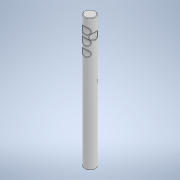
# Autodesk Inventor part: 79. Шток третьей и четвертой передач
Saved by Autodesk Inventor 2021 (Build 250183000, 183)
## iProperties
Created: 2021-03-18
Part Number: 79. Шток третьей и четвертой передач
Material: Типовые
Document SubType Name: Modeling
Designer: Данил
Density: 1 g/cm^3
Appearance: По умолчанию
Author: Данил
Autodesk Inventor part; units mm, degrees
ref_plane "YZ Plane" through (0, 0, 0) normal (1, 0, 0) x (0, 1, 0)
ref_plane "XZ Plane" through (0, 0, 0) normal (0, 1, 0) x (-1, 0, 0)
ref_plane "XY Plane" through (0, 0, 0) normal (0, 0, 1) x (1, 0, 0)
sketch "Эскиз1" plane through (0, 0, 0) normal (0, 0, 1) x (1, 0, 0)
  line L0 (0, 91.5) -> (0, -91.5)
  line L1 (0, -91.5) -> (6.75, -91.5)
  line L2 (7.5, -90.75) -> (7.5, 90.75)
  line L3 (6.75, 91.5) -> (0, 91.5)
  line L4 (7.5, -90.75) -> (6.75, -91.5)
  line L5 (7.5, 90.75) -> (6.75, 91.5)
  point P0 (0, 0)
  point P1 (0, 0)
  point P2 (7.5, -91.5)
  point P3 (7.5, 91.5)
  dimension "d0" = 183
  dimension "d1" = 15
  dimension "d2" = 0.75
  dimension "d3" = 45
  dimension "d4" = 0.75
  dimension "d5" = 45
  constraints: 12 end point, 4 point on line, 2 perpendicular, 1 coincident, 1 horizontal, 1 midpoint, 1 vertical
  measures "d0" distance of L0.start L0.end
  measures "d1" diameter of L2 L0
  measures "d2" distance of L2.start point (7.5, -91.5)
  measures "d3" angle of L2 L4
  measures "d4" distance of L2.end point (7.5, 91.5)
  measures "d5" angle of L2 L5
revolve "Вращение1" add sketch "Эскиз1" angle 360 about axis through (0, 91.5, 0) along (0, -1, 0)
sketch "Эскиз2" plane through (0, 0, 0) normal (1, 0, 0) x (0, 1, 0)
  line L0 (90.75, -7.5) -> (-90.75, -7.5) projected
  line L1 (90.75, 7.5) -> (-90.75, 7.5) projected
  line L2 (91.5, 6.75) -> (91.5, -6.75) projected
  arc A0 (71.1872, 7.5) -> (79.8128, 7.5) centre (75.5, 9.1) ccw
  arc A1 (57.6872, 7.5) -> (66.3128, 7.5) centre (62, 9.1) ccw
  arc A2 (44.1872, 7.5) -> (52.8128, 7.5) centre (48.5, 9.1) ccw
  point P0 (0, 0)
  point P1 (75.5, 4.5)
  point P2 (62, 4.5)
  point P3 (48.5, 4.5)
  point P4 (62, 4.5)
  point P5 (48.5, 4.5)
  dimension "d7" = 4.6
  dimension "d8" = 12
  dimension "d9" = 16
  dimension "d10" = 13.5
  dimension "d11" = 13.5
  constraints: 11 point on circle, 6 point on line, 4 horizontal alignment, 3 centre point, 3 vertical alignment
  measures "d7" radius of A0
  measures "d8" distance from line of L0 point (75.5, 4.5)
  measures "d9" distance from line of L2 A0.centre
  measures "d10" distance of A1.centre A0.centre
  measures "d11" distance of A2.centre A1.centre
extrude "Выдавливание1" cut sketch "Эскиз2" against normal through all both and the other way through all
ref_plane "РабПлоскость1" through (0, 10.75, 0) normal (0, 1, 0) x (1, 0, 0)
sketch "Эскиз3" plane through (0, 10.75, 0) normal (0, 1, 0) x (1, 0, 0)
  line L0 (2.0673, 7.2095) -> (-2.0673, -7.2095) construction
  circle A0 centre (0, 0) radius 7.5 projected
  line L1 (0, 0) -> (0, 7.5) construction
  point P0 (0, 0)
  point P1 (0, 0)
  dimension "d15" = 16
  constraints: 4 end point, 2 point on circle, 1 coincident, 1 midpoint, 1 vertical
  measures "d15" angle of L1 L0
ref_plane "РабПлоскость2" through (2.0673, 10.75, -7.2095) normal (-0.2756374, 0, 0.9612617) x (0, -1, 0)
hole "Отверстие1" at (2.0673, 10.75, -7.2095) direction (-0.2756374, 0, 0.9612617) diameter 4.5 depth 11 tip angle 120 countersink diameter 8.7 countersink angle 30
sketch "Эскиз4" plane through (0, 0, 0) normal (0, 0, 1) x (1, 0, 0)
  line L0 (7.5, 90.75) -> (7.5, -90.75) projected
  line L1 (-7.5, 90.75) -> (-7.5, -90.75) projected
  line L2 (-6.75, 91.5) -> (6.75, 91.5) projected
  arc A0 (7.5, 73.1997) -> (7.5, 64.3003) centre (9.3, 68.75) ccw
  ellipse E0 centre (-0.093, 10.75) end of major axis (-0.093, 8.5) minor radius 2.1628 projected
  point P0 (0, 0)
  point P1 (4.5, 68.75)
  dimension "d25" = 4.8
  dimension "d26" = 12
  dimension "d27" = 58
  constraints: 3 point on circle, 2 point on line, 1 centre point, 1 horizontal alignment
  measures "d25" radius of A0
  measures "d26" distance from line of L1 point (4.5, 68.75)
  measures "d27" vertical distance of A0.centre E0.centre
extrude "Выдавливание2" cut sketch "Эскиз4" along normal through all both and the other way through all contours L0 A0
mirror "Зеркальное отражение1" about plane through (0, 0, 0) normal (1, 0, 0) of "Выдавливание2"
fillet "Сопряжение1" radius 0.8 13 edges at (-4.2073, 79.0778, 6.2087) (-4.2054, 71.9212, 6.21) (6, 75.5001, 4.5) (-4.2073, 65.5778, 6.2087) (-4.2054, 58.4212, 6.21) (6, 62.0001, 4.5) (-4.2073, 52.0778, 6.2087) (-4.2054, 44.9212, 6.21) (6, 48.5001, 4.5) (4.5, 68.7507, -6) (4.5, 68.7507, 6) (-4.5, 68.7507, -6) (-4.5, 68.7507, 6)
equation "\"d4\" = d2"
equation "\"d5\" = d3"
